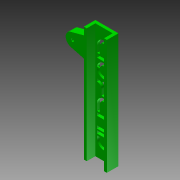
# Autodesk Inventor part: TabletMount-Mast-Left
Saved by Autodesk Inventor 2012 (Build 160160000, 160)
## iProperties
Created: 2013-10-06
Part Number: TabletMount-Mast-Left
Material: Default
Document SubType Name: Modeling
Designer: joe_000
Density: 1 g/cm^3
Author: joe_000
Autodesk Inventor part; units mm, degrees
ref_plane "YZ Plane" through (0, 0, 0) normal (1, 0, 0) x (0, 1, 0)
ref_plane "XZ Plane" through (0, 0, 0) normal (0, 1, 0) x (-1, 0, 0)
ref_plane "XY Plane" through (0, 0, 0) normal (0, 0, 1) x (1, 0, 0)
sketch "Sketch1" plane through (0, 0, 0) normal (0, 1, 0) x (-1, 0, 0)
  line L0 (0, 12.7) -> (0, 0)
  line L1 (0, 0) -> (25.4, 0)
  line L2 (25.4, 0) -> (25.4, 12.7)
  line L3 (25.4, 12.7) -> (22.225, 12.7)
  line L4 (22.225, 12.7) -> (22.225, 3.175)
  line L5 (22.225, 3.175) -> (3.175, 3.175)
  line L6 (3.175, 3.175) -> (3.175, 12.7)
  line L7 (3.175, 12.7) -> (0, 12.7)
  dimension "d0" = 19.05
  dimension "d1" = 3.175
  dimension "d2" = 3.175
  dimension "d3" = 3.175
  dimension "d4" = 9.525
  constraints: 16 end point, 5 parallel, 1 collinear, 1 horizontal, 1 perpendicular, 1 vertical
  measures "d0" distance of L4.end L5.end
  measures "d1" distance between parallel lines of L0 L6
  measures "d2" distance between parallel lines of L2 L4
  measures "d3" distance between parallel lines of L1 L5
  measures "d4" distance between parallel lines of L5 L3
extrude "Extrusion1" add sketch "Sketch1" along normal blind 127
sketch "Sketch3" plane through (0, 0, 0) normal (0, 0, -1) x (-1, 0, 0)
  line L0 (0, 0) -> (0, 127) projected
  line L1 (25.4, 0) -> (25.4, 127) projected
  line L2 (25.4, 115.4147) -> (44.45, 110.3102)
  line L3 (25.4, 90.8361) -> (44.45, 95.9406)
  arc A0 (44.45, 95.9406) -> (44.45, 110.3102) centre (42.5248, 103.1254) ccw
  point P0 (0, 115.8525)
  point P1 (0, 86.0657)
  dimension "d9" = 75
  dimension "d10" = 75
  dimension "d11" = 19.05
  dimension "d12" = 19.05
  constraints: 4 end point, 4 point on line, 2 point on circle, 1 centre point, 1 tangent
  measures "d9" angle of L1 L2
  measures "d10" angle of L1 L3
  measures "d11" horizontal distance of L2.start L2.end
  measures "d12" horizontal distance of L3.start L3.end
extrude "Extrusion2" add sketch "Sketch3" against normal blind 8.2127
hole "Hole1" at (-42.5248, 103.1254, 0) direction (0, 0, 1) diameter 3 end through all
fillet "Fillet1" radius 3.175 2 edges at (-25.4, 115.4147, 4.1063) (-25.4, 90.8361, 4.1063)
sketch "Sketch4" plane through (0, 0, 0) normal (0, 0, -1) x (-1, 0, 0)
  line L0 (5.1858, 10.3722) -> (5.1858, 116.7874) construction
  line L1 (5.1858, 116.7874) -> (20.4479, 116.7874) construction
  line L2 (20.4479, 116.7874) -> (20.4479, 10.3722) construction
  line L3 (20.4479, 10.3722) -> (5.1858, 10.3722) construction
  line L4 (5.1858, 18.6709) -> (5.1858, 25.7226)
  line L5 (5.1858, 25.7226) -> (20.4479, 25.7226)
  line L6 (20.4479, 25.7226) -> (20.4479, 22.6657)
  line L7 (20.4479, 22.6657) -> (8.1543, 22.6657)
  line L8 (8.1543, 22.6657) -> (8.1654, 19.9289)
  line L9 (8.1654, 19.9289) -> (8.1654, 19.2778)
  spline S0 degree 2 poles (8.1654, 19.2778) (8.1654, 16.9935) (8.353, 16.7397) knots 0 0 0 1 1 1
  spline S1 degree 2 poles (8.353, 16.7397) (8.7282, 15.3713) (9.931, 14.4222) knots 0 0 0 1 1 1
  spline S2 degree 2 poles (9.931, 14.4222) (11.3877, 13.407) (12.8223, 13.407) knots 0 0 0 1 1 1
  spline S3 degree 2 poles (12.8223, 13.407) (14.6101, 13.407) (16.0999, 14.7864) knots 0 0 0 1 1 1
  spline S4 degree 2 poles (16.0999, 14.7864) (16.9717, 15.7134) (17.1593, 16.3755) knots 0 0 0 1 1 1
  spline S5 degree 2 poles (17.1593, 16.3755) (17.4904, 17.0376) (17.4904, 18.6709) knots 0 0 0 1 1 1
  line L10 (17.4904, 18.6709) -> (17.4904, 20.8007)
  line L11 (17.4904, 20.8007) -> (20.4479, 20.8007)
  line L12 (20.4479, 20.8007) -> (20.4479, 18.2515)
  spline S6 degree 2 poles (20.4479, 18.2515) (20.4479, 15.4154) (18.9581, 13.4511) knots 0 0 0 1 1 1
  spline S7 degree 2 poles (18.9581, 13.4511) (17.8325, 12.0386) (16.9275, 11.553) knots 0 0 0 1 1 1
  spline S8 degree 2 poles (16.9275, 11.553) (15.0405, 10.3722) (13.0651, 10.3722) knots 0 0 0 1 1 1
  line L13 (13.0651, 10.3722) -> (12.6237, 10.3722)
  spline S9 degree 2 poles (12.6237, 10.3722) (9.8759, 10.3722) (7.5695, 12.4358) knots 0 0 0 1 1 1
  spline S10 degree 2 poles (7.5695, 12.4358) (6.3555, 13.6828) (6.0355, 14.4774) knots 0 0 0 1 1 1
  spline S11 degree 2 poles (6.0355, 14.4774) (5.7265, 15.0512) (5.4396, 16.0555) knots 0 0 0 1 1 1
  spline S12 degree 2 poles (5.4396, 16.0555) (5.1858, 16.9604) (5.1858, 18.6709) knots 0 0 0 1 1 1
  spline S13 degree 2 poles (5.2079, 35.0034) (5.2079, 38.6672) (8.2316, 41.1391) knots 0 0 0 1 1 1
  spline S14 degree 2 poles (8.2316, 41.1391) (8.8496, 41.5916) (9.28, 41.8013) knots 0 0 0 1 1 1
  spline S15 degree 2 poles (9.28, 41.8013) (9.7986, 42.0882) (10.6815, 42.353) knots 0 0 0 1 1 1
  spline S16 degree 2 poles (10.6815, 42.353) (11.7409, 42.6731) (13.5617, 42.6731) knots 0 0 0 1 1 1
  line L14 (13.5617, 42.6731) -> (20.4479, 42.6731)
  line L15 (20.4479, 42.6731) -> (20.4479, 39.6162)
  line L16 (20.4479, 39.6162) -> (13.2307, 39.6162)
  spline S17 degree 2 poles (13.2307, 39.6162) (9.5889, 39.6162) (8.353, 36.3277) knots 0 0 0 1 1 1
  spline S18 degree 2 poles (8.353, 36.3277) (8.1433, 35.5662) (8.1323, 35.0034) knots 0 0 0 1 1 1
  spline S19 degree 2 poles (8.1323, 35.0034) (8.1433, 34.4296) (8.353, 33.6902) knots 0 0 0 1 1 1
  spline S20 degree 2 poles (8.353, 33.6902) (9.5889, 30.3906) (13.2307, 30.3906) knots 0 0 0 1 1 1
  line L17 (13.2307, 30.3906) -> (20.4479, 30.3906)
  line L18 (20.4479, 30.3906) -> (20.4479, 27.3227)
  line L19 (20.4479, 27.3227) -> (13.5617, 27.3227)
  spline S21 degree 2 poles (13.5617, 27.3227) (11.7409, 27.3227) (10.6815, 27.6427) knots 0 0 0 1 1 1
  spline S22 degree 2 poles (10.6815, 27.6427) (9.7986, 27.9076) (9.28, 28.2055) knots 0 0 0 1 1 1
  spline S23 degree 2 poles (9.28, 28.2055) (8.8385, 28.4042) (8.2316, 28.8677) knots 0 0 0 1 1 1
  spline S24 degree 2 poles (8.2316, 28.8677) (5.2079, 31.3396) (5.2079, 35.0034) knots 0 0 0 1 1 1
  spline S25 degree 2 poles (5.1968, 49.7358) (5.1968, 52.8147) (5.3293, 53.2782) knots 0 0 0 1 1 1
  spline S26 degree 2 poles (5.3293, 53.2782) (5.4727, 54.5252) (6.3776, 56.0922) knots 0 0 0 1 1 1
  spline S27 degree 2 poles (6.3776, 56.0922) (6.9073, 56.9419) (7.9998, 57.9131) knots 0 0 0 1 1 1
  spline S28 degree 2 poles (7.9998, 57.9131) (10.1297, 59.6236) (12.8334, 59.6236) knots 0 0 0 1 1 1
  spline S29 degree 2 poles (12.8334, 59.6236) (14.4225, 59.6236) (15.835, 59.0166) knots 0 0 0 1 1 1
  spline S30 degree 2 poles (15.835, 59.0166) (18.5718, 57.8027) (19.7968, 55.0438) knots 0 0 0 1 1 1
  spline S31 degree 2 poles (19.7968, 55.0438) (20.4479, 53.7637) (20.4479, 51.1042) knots 0 0 0 1 1 1
  line L20 (20.4479, 51.1042) -> (20.4479, 44.6153)
  line L21 (20.4479, 44.6153) -> (20.3816, 44.2732)
  line L22 (20.3816, 44.2732) -> (17.4904, 44.2732)
  line L23 (17.4904, 44.2732) -> (17.4904, 51.4352)
  spline S32 degree 2 poles (17.4904, 51.4352) (17.4904, 52.5719) (17.2807, 53.2009) knots 0 0 0 1 1 1
  spline S33 degree 2 poles (17.2807, 53.2009) (16.7179, 54.8562) (15.6143, 55.6397) knots 0 0 0 1 1 1
  spline S34 degree 2 poles (15.6143, 55.6397) (14.2018, 56.5778) (12.8665, 56.5778) knots 0 0 0 1 1 1
  spline S35 degree 2 poles (12.8665, 56.5778) (11.5202, 56.5778) (10.218, 55.7611) knots 0 0 0 1 1 1
  spline S36 degree 2 poles (10.218, 55.7611) (9.4676, 55.2535) (9.0813, 54.6355) knots 0 0 0 1 1 1
  spline S37 degree 2 poles (9.0813, 54.6355) (8.1543, 53.5209) (8.1543, 51.4352) knots 0 0 0 1 1 1
  line L24 (8.1543, 51.4352) -> (8.1543, 44.2732)
  line L25 (8.1543, 44.2732) -> (5.1968, 44.2732)
  line L26 (5.1968, 44.2732) -> (5.1968, 49.7358)
  line L27 (5.1968, 61.2237) -> (5.1968, 71.0232)
  spline S38 degree 2 poles (5.1968, 71.0232) (5.1968, 73.6276) (6.7528, 75.0953) knots 0 0 0 1 1 1
  spline S39 degree 2 poles (6.7528, 75.0953) (7.3598, 75.7464) (7.9336, 76.0002) knots 0 0 0 1 1 1
  spline S40 degree 2 poles (7.9336, 76.0002) (9.0813, 76.5741) (10.1738, 76.5741) knots 0 0 0 1 1 1
  line L28 (10.1738, 76.5741) -> (10.6042, 76.5741)
  spline S41 degree 2 poles (10.6042, 76.5741) (12.2706, 76.5741) (13.8707, 75.1284) knots 0 0 0 1 1 1
  spline S42 degree 2 poles (13.8707, 75.1284) (14.7646, 74.1904) (15.0184, 73.4289) knots 0 0 0 1 1 1
  spline S43 degree 2 poles (15.0184, 73.4289) (17.071, 75.3602) (20.4479, 75.3602) knots 0 0 0 1 1 1
  line L29 (20.4479, 75.3602) -> (20.4479, 72.2813)
  line L30 (20.4479, 72.2813) -> (20.2161, 72.2813)
  spline S44 degree 2 poles (20.2161, 72.2813) (17.7221, 72.2813) (16.2433, 70.2507) knots 0 0 0 1 1 1
  spline S45 degree 2 poles (16.2433, 70.2507) (15.4267, 69.103) (15.4267, 67.238) knots 0 0 0 1 1 1
  line L31 (15.4267, 67.238) -> (15.4267, 61.2237)
  line L32 (15.4267, 61.2237) -> (12.4913, 61.2237)
  line L33 (12.4913, 61.2237) -> (12.4913, 71.2218)
  spline S46 degree 2 poles (12.4913, 71.2218) (12.4913, 72.8551) (10.8691, 73.44) knots 0 0 0 1 1 1
  spline S47 degree 2 poles (10.8691, 73.44) (10.538, 73.5062) (10.3173, 73.5283) knots 0 0 0 1 1 1
  spline S48 degree 2 poles (10.3173, 73.5283) (9.4124, 73.5283) (8.684, 72.7778) knots 0 0 0 1 1 1
  spline S49 degree 2 poles (8.684, 72.7778) (8.1764, 72.1268) (8.1764, 71.3984) knots 0 0 0 1 1 1
  spline S50 degree 2 poles (8.1764, 71.3984) (8.1323, 71.3984) (8.1323, 70.957) knots 0 0 0 1 1 1
  line L34 (8.1323, 70.957) -> (8.1323, 61.2237)
  line L35 (8.1323, 61.2237) -> (5.1968, 61.2237)
  line L36 (5.2079, 85.8108) -> (5.2079, 85.9101)
  spline S51 degree 2 poles (5.2079, 85.9101) (5.2079, 89.4304) (8.0881, 91.9134) knots 0 0 0 1 1 1
  spline S52 degree 2 poles (8.0881, 91.9134) (10.24, 93.5246) (12.7892, 93.5246) knots 0 0 0 1 1 1
  line L37 (12.7892, 93.5246) -> (12.8886, 93.5246)
  spline S53 degree 2 poles (12.8886, 93.5246) (16.4089, 93.5246) (18.8588, 90.5891) knots 0 0 0 1 1 1
  spline S54 degree 2 poles (18.8588, 90.5891) (20.4479, 88.4482) (20.4479, 85.888) knots 0 0 0 1 1 1
  line L38 (20.4479, 85.888) -> (20.4479, 85.7887)
  spline S55 degree 2 poles (20.4479, 85.7887) (20.4479, 82.2904) (17.5897, 79.8075) knots 0 0 0 1 1 1
  spline S56 degree 2 poles (17.5897, 79.8075) (16.3758, 78.9356) (15.3605, 78.5825) knots 0 0 0 1 1 1
  spline S57 degree 2 poles (15.3605, 78.5825) (14.0914, 78.1742) (12.8665, 78.1742) knots 0 0 0 1 1 1
  line L39 (12.8665, 78.1742) -> (12.7672, 78.1742)
  spline S58 degree 2 poles (12.7672, 78.1742) (9.3131, 78.1742) (6.8521, 81.0214) knots 0 0 0 1 1 1
  spline S59 degree 2 poles (6.8521, 81.0214) (5.4727, 82.9526) (5.3072, 84.5417) knots 0 0 0 1 1 1
  spline S60 degree 2 poles (5.3072, 84.5417) (5.2079, 85.0272) (5.2079, 85.8108) knots 0 0 0 1 1 1
  spline S61 degree 2 poles (12.8003, 81.22) (14.7977, 81.22) (16.2985, 82.776) knots 0 0 0 1 1 1
  spline S62 degree 2 poles (16.2985, 82.776) (17.4904, 84.1665) (17.4904, 85.6894) knots 0 0 0 1 1 1
  line L40 (17.4904, 85.6894) -> (17.4904, 85.9873)
  spline S63 degree 2 poles (17.4904, 85.9873) (17.4904, 87.2123) (16.6517, 88.4924) knots 0 0 0 1 1 1
  spline S64 degree 2 poles (16.6517, 88.4924) (15.6805, 89.8056) (14.1907, 90.2691) knots 0 0 0 1 1 1
  spline S65 degree 2 poles (14.1907, 90.2691) (13.8045, 90.4125) (12.8444, 90.4788) knots 0 0 0 1 1 1
  spline S66 degree 2 poles (12.8444, 90.4788) (10.9022, 90.4788) (9.4013, 88.9669) knots 0 0 0 1 1 1
  spline S67 degree 2 poles (9.4013, 88.9669) (8.1433, 87.5433) (8.1433, 85.8549) knots 0 0 0 1 1 1
  spline S68 degree 2 poles (8.1433, 85.8549) (8.1433, 83.8685) (9.7986, 82.3346) knots 0 0 0 1 1 1
  spline S69 degree 2 poles (9.7986, 82.3346) (10.6484, 81.6945) (11.2332, 81.518) knots 0 0 0 1 1 1
  spline S70 degree 2 poles (11.2332, 81.518) (12.0609, 81.22) (12.8003, 81.22) knots 0 0 0 1 1 1
  line L41 (5.2079, 95.1247) -> (5.2079, 98.1815)
  line L42 (5.2079, 98.1815) -> (20.4479, 98.1815)
  line L43 (20.4479, 98.1815) -> (20.4479, 95.1247)
  line L44 (20.4479, 95.1247) -> (5.2079, 95.1247)
  spline S71 degree 2 poles (5.1968, 105.2994) (5.1968, 108.3783) (5.3293, 108.8418) knots 0 0 0 1 1 1
  spline S72 degree 2 poles (5.3293, 108.8418) (5.4727, 110.0888) (6.3776, 111.6559) knots 0 0 0 1 1 1
  spline S73 degree 2 poles (6.3776, 111.6559) (6.9073, 112.5056) (7.9998, 113.4767) knots 0 0 0 1 1 1
  spline S74 degree 2 poles (7.9998, 113.4767) (10.1297, 115.1872) (12.8334, 115.1872) knots 0 0 0 1 1 1
  spline S75 degree 2 poles (12.8334, 115.1872) (14.4225, 115.1872) (15.835, 114.5803) knots 0 0 0 1 1 1
  spline S76 degree 2 poles (15.835, 114.5803) (18.5718, 113.3664) (19.7968, 110.6075) knots 0 0 0 1 1 1
  spline S77 degree 2 poles (19.7968, 110.6075) (20.4479, 109.3274) (20.4479, 106.6678) knots 0 0 0 1 1 1
  line L45 (20.4479, 106.6678) -> (20.4479, 100.179)
  line L46 (20.4479, 100.179) -> (20.3816, 99.8369)
  line L47 (20.3816, 99.8369) -> (17.4904, 99.8369)
  line L48 (17.4904, 99.8369) -> (17.4904, 106.9989)
  spline S78 degree 2 poles (17.4904, 106.9989) (17.4904, 108.1355) (17.2807, 108.7646) knots 0 0 0 1 1 1
  spline S79 degree 2 poles (17.2807, 108.7646) (16.7179, 110.4199) (15.6143, 111.2034) knots 0 0 0 1 1 1
  spline S80 degree 2 poles (15.6143, 111.2034) (14.2018, 112.1414) (12.8665, 112.1414) knots 0 0 0 1 1 1
  spline S81 degree 2 poles (12.8665, 112.1414) (11.5202, 112.1414) (10.218, 111.3248) knots 0 0 0 1 1 1
  spline S82 degree 2 poles (10.218, 111.3248) (9.4676, 110.8172) (9.0813, 110.1992) knots 0 0 0 1 1 1
  spline S83 degree 2 poles (9.0813, 110.1992) (8.1543, 109.0846) (8.1543, 106.9989) knots 0 0 0 1 1 1
  line L49 (8.1543, 106.9989) -> (8.1543, 99.8369)
  line L50 (8.1543, 99.8369) -> (5.1968, 99.8369)
  line L51 (5.1968, 99.8369) -> (5.1968, 105.2994)
  constraints: 2 other
extrude "Extrusion3" cut sketch "Sketch4" against normal up to next
sketch "Sketch5" plane through (-17.4904, 85.6894, 3.175) normal (0, 0, 1) x (1, 0, 0)
  line L0 (-3.4862, 0.9233) -> (13.018, 0.9233)
  line L1 (13.018, 0.9233) -> (13.018, -0.7757)
  line L2 (13.018, -0.7757) -> (-3.4862, -0.7757)
  line L3 (-3.4862, -0.7757) -> (-3.4862, 0.9233)
  point P0 (17.4904, -85.6894)
  constraints: 8 end point, 2 parallel, 1 horizontal, 1 perpendicular
extrude "Extrusion4" add sketch "Sketch5" against normal blind 1.27
equation "\"d0\" = MastWidth"
equation "\"d1\" = WallThickness"
equation "\"d2\" = WallThickness"
equation "\"d3\" = WallThickness"
equation "\"d4\" = 0.5 * MastWidth"
equation "\"d5\" = Length"
equation "\"d9\" = HingeAngle"
equation "\"d10\" = HingeAngle"
equation "\"d11\" = HingeLength"
equation "\"d12\" = HingeLength"
equation "\"d13\" = HingeHoleDiameter"
equation "\"MastWidth\" = 19.05"
equation "\"WallThickness\" = 3.175"
equation "\"Length\" = 127"
equation "\"HingeAngle\" = 75deg"
equation "\"HingeLength\" = 19.05"
equation "\"HingeHoleDiameter\" = 3"
body "Solid1"
